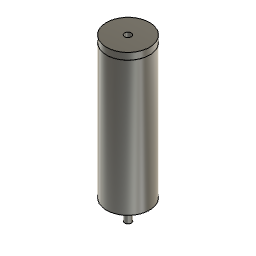
seal_chamber (Autodesk Fusion 360 design; units mm, degrees)
Autodesk Fusion 360 part; units mm, degrees
note: some values were not read from the file. Set by a fixed rule: which sketch regions a step uses.
sketch "Sketch1" plane through (0, 0, 0) normal (0, 0, 1) x (1, 0, 0)
  circle A0 centre (0, 0) radius 7.5
  circle A1 centre (0, 0) radius 2.6
  circle A2 centre (0, 0) radius 16
  circle A3 centre (0, 0) radius 12.625
  circle A4 centre (0, 0) radius 8
  line L0 (0, 0) -> (0, 12.625) construction
  line L1 (0, 12.625) -> (0, 8.625) construction
  line L2 (0, 0) -> (-12.625, 0) construction
  circle A5 centre (0, 0) radius 5
  circle A6 centre (0, 0) radius 6.75
  dimension "d1" = 15
  dimension "d2" = 5.2
  dimension "d3" = 32
  dimension "d4" = 25.25
  dimension "d10" = 16
  dimension "d13" = 4
  dimension "d26" = 10
  dimension "d27" = 13.5
  constraint coincident A0.centre A1.centre
  constraint concentric A0 A1
  constraint concentric A0 A2
  constraint concentric A2 A3
  constraint concentric A0 A4
  constraint coincident A3 L0.end
  constraint vertical L0
  constraint coincident L0 L1.end
  constraint coincident A3 L2.end
  constraint perpendicular L0 L2
  constraint concentric A4 A5
  constraint concentric A2 A6
  measures "d1" diameter of A0
  measures "d2" diameter of A1
  measures "d3" diameter of A2
  measures "d4" diameter of A3
  measures "d10" diameter of A4
  measures "d13" distance of L0.end L1.end
  measures "d26" diameter of A5
  measures "d27" diameter of A6
extrude "Extrude1" add sketch "Sketch1" along normal blind 6 contours A3 | A4 makes body 1
extrude "Extrude2" add sketch "Sketch1" along normal blind 10 from surface at 6 contours A0 | A3 | A4 | A5 | A6 bodies 1
extrude "Extrude6" add sketch "Sketch1" against normal blind 2.5 from surface at 6 contours A6 bodies 1
extrude "Extrude7" cut sketch "Sketch1" against normal blind 5.3 from surface at 16 contours A0 | A4 | A5 | A6 bodies 1
extrude "Extrude3" add sketch "Sketch1" along normal blind 100 contours A2 bodies 1
sketch "Sketch2" plane through (0, 0, 0) normal (0, 0, 1) x (1, 0, 0)
  circle A0 centre (0, 0) radius 2.5
  circle A1 centre (0, 0) radius 16.031
  dimension "d34" = 5
  constraint coincident A0.centre A1.centre
  measures "d34" diameter of A0
extrude "Extrude8" add sketch "Sketch2" along normal blind 5 separate body makes body 2
extrude "Extrude9" add sketch "Sketch2" against normal blind 115 contours A0 bodies 2
move_body "Move1" bodies 2 to x (1, 0, 0) y (0, 1, 0) z (0, 0, 1) at (0, 0, 100)
equation "d11 = 16 mm + 84 mm"
